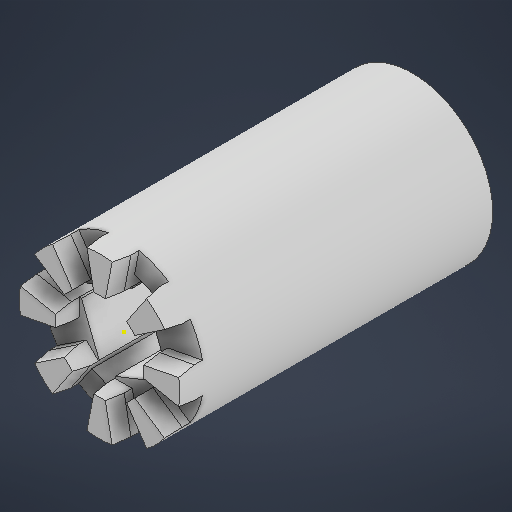
# Autodesk Inventor part: деталь вв
Saved by Autodesk Inventor 2025 (Build 290162000, 162)
## iProperties
Created: 2024-11-26
Part Number: деталь вв
Material: Типовые
Document SubType Name: Modeling
Designer: Phantom
Density: 1 g/cm^3
Appearance: По умолчанию
Author: Phantom
Autodesk Inventor part; units mm, degrees
ref_plane "YZ Plane" through (0, 0, 0) normal (1, 0, 0) x (0, 1, 0)
ref_plane "XZ Plane" through (0, 0, 0) normal (0, 1, 0) x (-1, 0, 0)
ref_plane "XY Plane" through (0, 0, 0) normal (0, 0, 1) x (1, 0, 0)
sketch "Эскиз1" plane through (0, 0, 0) normal (0, 0, 1) x (1, 0, 0)
  circle A0 centre (0, 0) radius 10
  line L0 (-3.8095, 3.8095) -> (3.8095, 3.8095)
  line L1 (3.8095, 3.8095) -> (3.8095, -3.8095)
  line L2 (3.8095, -3.8095) -> (-3.8095, -3.8095)
  line L3 (-3.8095, -3.8095) -> (-3.8095, 3.8095)
  line L4 (-3.8095, 3.8095) -> (3.8095, -3.8095) construction
  line L5 (3.8095, 3.8095) -> (-3.8095, -3.8095) construction
  dimension "d0" = 20
  constraints: 12 end point, 2 midpoint, 2 parallel, 1 centre point, 1 coincident, 1 horizontal, 1 perpendicular
  measures "d0" diameter of A0
extrude "Выдавливание1" add sketch "Эскиз1" along normal blind 36
sketch "Эскиз2" plane through (0, 0, 36) normal (0, 0, 1) x (1, 0, 0)
  line L0 (-3.8095, 3.8095) -> (3.8095, 3.8095) projected
  circle A0 centre (0, 0) radius 10 projected
  line L1 (9.8151, 1.914) -> (5.5, 1.0725)
  line L2 (5.5, -1.0775) -> (9.8135, -1.9225)
  line L3 (5.5, 0) -> (5.5, 1.0725)
  line L4 (5.5, 1.0725) -> (5.5, -1.0775)
  line L5 (5.587, 8.2937) -> (3.1307, 4.6475)
  line L6 (4.651, 3.1272) -> (8.2986, 5.5797)
  line L7 (3.8891, 3.8891) -> (3.1307, 4.6475)
  line L8 (3.1307, 4.6475) -> (4.651, 3.1272)
  line L9 (-1.914, 9.8151) -> (-1.0725, 5.5)
  line L10 (1.0775, 5.5) -> (1.9225, 9.8135)
  line L11 (0, 5.5) -> (-1.0725, 5.5)
  line L12 (-1.0725, 5.5) -> (1.0775, 5.5)
  line L13 (-8.2937, 5.587) -> (-4.6475, 3.1307)
  line L14 (-3.1272, 4.651) -> (-5.5797, 8.2986)
  line L15 (-3.8891, 3.8891) -> (-4.6475, 3.1307)
  line L16 (-4.6475, 3.1307) -> (-3.1272, 4.651)
  line L17 (-9.8151, -1.914) -> (-5.5, -1.0725)
  line L18 (-5.5, 1.0775) -> (-9.8135, 1.9225)
  line L19 (-5.5, 0) -> (-5.5, -1.0725)
  line L20 (-5.5, -1.0725) -> (-5.5, 1.0775)
  line L21 (-5.587, -8.2937) -> (-3.1307, -4.6475)
  line L22 (-4.651, -3.1272) -> (-8.2986, -5.5797)
  line L23 (-3.8891, -3.8891) -> (-3.1307, -4.6475)
  line L24 (-3.1307, -4.6475) -> (-4.651, -3.1272)
  line L25 (1.914, -9.8151) -> (1.0725, -5.5)
  line L26 (-1.0775, -5.5) -> (-1.9225, -9.8135)
  line L27 (0, -5.5) -> (1.0725, -5.5)
  line L28 (1.0725, -5.5) -> (-1.0775, -5.5)
  line L29 (8.2937, -5.587) -> (4.6475, -3.1307)
  line L30 (3.1272, -4.651) -> (5.5797, -8.2986)
  line L31 (3.8891, -3.8891) -> (4.6475, -3.1307)
  line L32 (4.6475, -3.1307) -> (3.1272, -4.651)
  dimension "d36" = 360
  constraints: 64 end point, 2 point on circle, 73 other
extrude "Выдавливание2" add sketch "Эскиз2" along normal blind 3 contours A0 L2 L4 L3 L1 | L6 L8 L7 L5 A0 | A0 L30 L32 L31 L29 | L10 L12 L11 L9 A0 | A0 L26 L28 L27 L25 | L14 L16 L15 L13 A0 | A0 L22 L24 L23 L21 | L18 L20 L19 L17 A0
chamfer "Фаска1" distance 2 angle 10 1 edges at (4.3588, 6.4706, 39) measured on face at (4.7682, 7.0783, 37)
chamfer "Фаска2" distance 2 angle 10 1 edges at (6.4748, 4.3535, 39) measured on face at (5.8669, 3.9447, 37)
chamfer "Фаска3" distance 2 angle 10 1 edges at (7.6576, 1.4932, 39) measured on face at (8.3768, 1.6335, 37)
chamfer "Фаска4" distance 2 angle 10 1 edges at (7.6567, -1.5, 39) measured on face at (6.9378, -1.3592, 37)
chamfer "Фаска5" distance 2 angle 10 1 edges at (6.4706, -4.3588, 39) measured on face at (7.0783, -4.7682, 37)
chamfer "Фаска6" distance 2 angle 10 1 edges at (4.3535, -6.4748, 39) measured on face at (3.9447, -5.8669, 37)
chamfer "Фаска7" distance 2 angle 10 1 edges at (-1.5, -7.6567, 39) measured on face at (-1.3592, -6.9378, 37)
chamfer "Фаска8" distance 2 angle 10 1 edges at (1.4932, -7.6576, 39) measured on face at (1.6335, -8.3768, 37)
chamfer "Фаска9" distance 2 angle 10 1 edges at (-6.4748, -4.3535, 39) measured on face at (-5.8669, -3.9447, 37)
chamfer "Фаска10" distance 2 angle 10 1 edges at (-4.3588, -6.4706, 39) measured on face at (-4.7682, -7.0783, 37)
chamfer "Фаска11" distance 2 angle 10 1 edges at (-7.6567, 1.5, 39) measured on face at (-6.9378, 1.3592, 37)
chamfer "Фаска12" distance 2 angle 10 1 edges at (-7.6576, -1.4932, 39) measured on face at (-8.3768, -1.6335, 37)
chamfer "Фаска13" distance 2 angle 10 1 edges at (-4.3535, 6.4748, 39) measured on face at (-3.9447, 5.8669, 37)
chamfer "Фаска14" distance 2 angle 10 1 edges at (-6.4706, 4.3588, 39) measured on face at (-7.0783, 4.7682, 37)
chamfer "Фаска15" distance 2 angle 10 1 edges at (1.5, 7.6567, 39) measured on face at (1.3592, 6.9378, 37)
chamfer "Фаска16" distance 2 angle 10 1 edges at (-1.4932, 7.6576, 39) measured on face at (-1.6335, 8.3768, 37)
sketch "Эскиз3" plane through (0, 0, 36) normal (0, 0, 1) x (1, 0, 0)
  point P0 (0, 0)
sketch "Эскиз5" plane through (0, 0, 36) normal (0, 0, 1) x (1, 0, 0)
  point P0 (0, 0)
sketch "Эскиз6" plane through (0, 0, 36) normal (0, 0, 1) x (1, 0, 0)
  line L0 (-1.0725, 5.5) -> (-1.914, 9.8151) projected
  arc A0 (-1.914, 9.8151) -> (-5.5797, 8.2986) centre (0, 0) ccw projected
  line L1 (-5.5797, 8.2986) -> (-3.1272, 4.651) projected
  line L2 (-3.1272, 4.651) -> (-4.6475, 3.1307) projected
  line L3 (-4.6475, 3.1307) -> (-8.2937, 5.587) projected
  arc A1 (-8.2937, 5.587) -> (-9.8135, 1.9225) centre (0, 0) ccw projected
  line L4 (-9.8135, 1.9225) -> (-5.5, 1.0775) projected
  line L5 (-5.5, 1.0775) -> (-5.5, -1.0725) projected
  line L6 (-5.5, -1.0725) -> (-9.8151, -1.914) projected
  arc A2 (-9.8151, -1.914) -> (-8.2986, -5.5797) centre (0, 0) ccw projected
  line L7 (-8.2986, -5.5797) -> (-4.651, -3.1272) projected
  line L8 (-4.651, -3.1272) -> (-3.1307, -4.6475) projected
  line L9 (-3.1307, -4.6475) -> (-5.587, -8.2937) projected
  arc A3 (-5.587, -8.2937) -> (-1.9225, -9.8135) centre (0, 0) ccw projected
  line L10 (-1.9225, -9.8135) -> (-1.0775, -5.5) projected
  line L11 (-1.0775, -5.5) -> (1.0725, -5.5) projected
  line L12 (1.0725, -5.5) -> (1.914, -9.8151) projected
  arc A4 (1.914, -9.8151) -> (5.5797, -8.2986) centre (0, 0) ccw projected
  line L13 (5.5797, -8.2986) -> (3.1272, -4.651) projected
  line L14 (3.1272, -4.651) -> (4.6475, -3.1307) projected
  line L15 (4.6475, -3.1307) -> (8.2937, -5.587) projected
  arc A5 (8.2937, -5.587) -> (9.8135, -1.9225) centre (0, 0) ccw projected
  line L16 (9.8135, -1.9225) -> (5.5, -1.0775) projected
  line L17 (5.5, -1.0775) -> (5.5, 1.0725) projected
  line L18 (5.5, 1.0725) -> (9.8151, 1.914) projected
  arc A6 (9.8151, 1.914) -> (8.2986, 5.5797) centre (0, 0) ccw projected
  line L19 (8.2986, 5.5797) -> (4.651, 3.1272) projected
  line L20 (4.651, 3.1272) -> (3.1307, 4.6475) projected
  line L21 (3.1307, 4.6475) -> (5.587, 8.2937) projected
  arc A7 (5.587, 8.2937) -> (1.9225, 9.8135) centre (0, 0) ccw projected
  line L22 (1.9225, 9.8135) -> (1.0775, 5.5) projected
  line L23 (1.0775, 5.5) -> (-1.0725, 5.5) projected
  line L24 (-3.8095, 3.8095) -> (3.8095, 3.8095) projected
  line L25 (3.8095, 3.8095) -> (3.8095, -3.8095) projected
  line L26 (3.8095, -3.8095) -> (-3.8095, -3.8095) projected
  line L27 (-3.8095, -3.8095) -> (-3.8095, 3.8095) projected
extrude "Выдавливание4" add sketch "Эскиз6" against normal up to surface (36 mm away) contours L24 L25 L26 L27
sketch "Эскиз7" plane through (0, 0, 36) normal (0, 0, 1) x (1, 0, 0)
  line L0 (-5.8493, 2.507) -> (2.507, 5.8493)
  line L1 (2.507, 5.8493) -> (5.8493, -2.507)
  line L2 (5.8493, -2.507) -> (-2.507, -5.8493)
  line L3 (-2.507, -5.8493) -> (-5.8493, 2.507)
  line L4 (-5.8493, 2.507) -> (5.8493, -2.507) construction
  line L5 (2.507, 5.8493) -> (-2.507, -5.8493) construction
  point P0 (0, 0)
  dimension "d95" = 9
  dimension "d96" = 9
  constraints: 12 end point, 2 parallel, 1 perpendicular
  measures "d95" distance of L1.end L2.end
  measures "d96" distance of L0.end L1.end
extrude "Выдавливание5" cut sketch "Эскиз7" against normal through all
sketch "Эскиз8" plane through (0, 0, 36) normal (0, 0, 1) x (1, 0, 0)
  line L0 (-4.651, -3.1272) -> (-3.1307, -4.6475) projected
  line L1 (-1.0775, -5.5) -> (1.0725, -5.5) projected
  line L2 (-3.1307, -4.6475) -> (-1.0775, -5.5)
  line L3 (-1.0775, -5.5) -> (-1.3659, -6.972)
  line L4 (-1.9225, -9.8135) -> (-1.0775, -5.5) projected
  line L5 (-3.1307, -4.6475) -> (-3.9688, -5.8915)
  line L6 (-3.1307, -4.6475) -> (-5.587, -8.2937) projected
  line L7 (-3.9688, -5.8915) -> (-1.3659, -6.972)
  line L8 (4.6475, -3.1307) -> (5.8915, -3.9688)
  line L9 (5.5, -1.0775) -> (6.972, -1.3659)
  line L10 (4.6475, -3.1307) -> (5.5, -1.0775)
  line L11 (5.8915, -3.9688) -> (6.972, -1.3659)
  line L12 (3.1307, 4.6475) -> (3.9688, 5.8915)
  line L13 (1.0775, 5.5) -> (1.3659, 6.972)
  line L14 (3.1307, 4.6475) -> (1.0775, 5.5)
  line L15 (3.9688, 5.8915) -> (1.3659, 6.972)
  line L16 (-4.6475, 3.1307) -> (-5.8915, 3.9688)
  line L17 (-5.5, 1.0775) -> (-6.972, 1.3659)
  line L18 (-4.6475, 3.1307) -> (-5.5, 1.0775)
  line L19 (-5.8915, 3.9688) -> (-6.972, 1.3659)
  point P0 (0, 0)
  dimension "d99" = 1.5
  dimension "d100" = 1.5
  dimension "d103" = 360
  constraints: 32 end point, 2 point on line, 33 other
  measures "d99" distance of L1.start L3.end
  measures "d100" distance of L0.end L5.end
extrude "Выдавливание6" cut sketch "Эскиз8" against normal through all
sketch "Эскиз9" plane through (0, 0, 36) normal (0, 0, 1) x (1, 0, 0)
  line L0 (-1.3659, -6.972) -> (-1.0775, -5.5) projected
  line L1 (-1.0775, -5.5) -> (-1, -5)
  line L2 (-3.1307, -4.6475) -> (-3.9688, -5.8915) projected
  line L3 (-3.1307, -4.6475) -> (-2.4444, -3.6286)
  line L4 (-2.4444, -3.6286) -> (-1, -5)
  line L5 (-3.1307, -4.6475) -> (-1.0775, -5.5)
  line L6 (5.5, -1.0775) -> (5, -1)
  line L7 (4.6475, -3.1307) -> (3.6286, -2.4444)
  line L8 (3.6286, -2.4444) -> (5, -1)
  line L9 (4.6475, -3.1307) -> (5.5, -1.0775)
  line L10 (1.0775, 5.5) -> (1, 5)
  line L11 (3.1307, 4.6475) -> (2.4444, 3.6286)
  line L12 (2.4444, 3.6286) -> (1, 5)
  line L13 (3.1307, 4.6475) -> (1.0775, 5.5)
  line L14 (-5.5, 1.0775) -> (-5, 1)
  line L15 (-4.6475, 3.1307) -> (-3.6286, 2.4444)
  line L16 (-3.6286, 2.4444) -> (-5, 1)
  line L17 (-4.6475, 3.1307) -> (-5.5, 1.0775)
  point P0 (0, 0)
  dimension "d109" = 360
  constraints: 32 end point, 1 collinear, 33 other
extrude "Выдавливание7" cut sketch "Эскиз9" against normal through all
